Autodesk Fusion 360 part; units mm, degrees
note: some values were not read from the file. Set by a fixed rule: which sketch regions a step uses.
(part 2 of 2)
extrude "Extruir44" add sketch "Boceto37" along normal blind 1 bodies 7
mirror "Simetría3" about plane through (0, 238.5, 45.4) normal (1, 0, 0) of bodies 7 merged
sketch "Boceto38" plane through (0, 266.5, 0) normal (0, 1, 0) x (-1, 0, 0)
  line L0 (-75, 1.5333) -> (-75, 8.4667)
  line L1 (-75, 8.4667) -> (-88.0667, 8.4667)
  line L2 (-88.0667, 8.4667) -> (-88.0667, 1.5333)
  line L3 (-88.0667, 1.5333) -> (-75, 1.5333)
sketch "Boceto44" plane through (88.0667, 0, 0) normal (1, 0, 0) x (0, 1, 0)
  line L0 (189.5, 8.4667) -> (189.5, 1.5333)
  line L1 (189.5, 1.5333) -> (266.5, 1.5333)
  line L2 (266.5, 1.5333) -> (266.5, 8.4667)
  line L3 (266.5, 8.4667) -> (189.5, 8.4667)
  line L4 (266.5, 8.4667) -> (184.5, 8.4667)
  line L5 (184.5, 8.4667) -> (184.5, 7.9667)
  line L6 (184.5, 7.9667) -> (266.5, 7.9667)
  line L7 (266.5, 7.9667) -> (266.5, 8.4667)
  line L8 (266.5, 1.5333) -> (184.5, 1.5333)
  line L9 (184.5, 1.5333) -> (184.5, 2.0333)
  line L10 (184.5, 2.0333) -> (266.5, 2.0333)
  line L11 (266.5, 2.0333) -> (266.5, 1.5333)
  dimension "d231" = 82
  dimension "d232" = 0.5
  dimension "d233" = 82
  dimension "d234" = 0.5
  constraint horizontal L4
  constraint vertical L5
  constraint horizontal L6
  constraint vertical L7
  constraint coincident L2.end L3.start
  constraint horizontal L8
  constraint vertical L9
  constraint horizontal L10
  constraint vertical L11
  constraint coincident L1.end L2.start
  measures "d231" distance of L2.end L4.end
  measures "d232" distance of L2.end L6.end
  measures "d233" distance of L1.end L8.end
  measures "d234" distance of L1.end L10.end
extrude "Extruir48" cut sketch "Boceto44" against normal blind 13.067 contours L0 L2 L3 L4 L6 L7 | L0 L4 L5 L6 | L0 L1 L2 L8 L10 L11 | L0 L8 L9 L10 bodies 3
sketch "Boceto45" plane through (-88.0667, 0, 0) normal (-1, 0, 0) x (0, -1, 0)
  line L0 (-189.5, 1.5333) -> (-189.5, 8.4667)
  line L1 (-189.5, 8.4667) -> (-266.5, 8.4667)
  line L2 (-266.5, 8.4667) -> (-266.5, 1.5333)
  line L3 (-266.5, 1.5333) -> (-189.5, 1.5333)
  line L4 (-266.5, 1.5333) -> (-184.5, 1.5333)
  line L5 (-184.5, 1.5333) -> (-184.5, 2.0333)
  line L6 (-184.5, 2.0333) -> (-266.5, 2.0333)
  line L7 (-266.5, 2.0333) -> (-266.5, 1.5333)
  line L8 (-266.5, 8.4667) -> (-184.5, 8.4667)
  line L9 (-184.5, 8.4667) -> (-184.5, 7.9667)
  line L10 (-184.5, 7.9667) -> (-266.5, 7.9667)
  line L11 (-266.5, 7.9667) -> (-266.5, 8.4667)
  dimension "d237" = 82
  dimension "d238" = 0.5
  dimension "d239" = 82
  dimension "d240" = 0.5
  constraint horizontal L4
  constraint vertical L5
  constraint horizontal L6
  constraint vertical L7
  constraint coincident L2.end L3.start
  constraint horizontal L8
  constraint vertical L9
  constraint horizontal L10
  constraint vertical L11
  constraint coincident L1.end L2.start
  measures "d237" distance of L2.end L4.end
  measures "d238" distance of L2.end L6.end
  measures "d239" distance of L1.end L8.end
  measures "d240" distance of L1.end L10.end
extrude "Extruir49" cut sketch "Boceto45" against normal blind 13.067 contours L0 L2 L3 L4 L6 L7 | L0 L4 L5 L6 | L0 L1 L2 L8 L10 L11 | L0 L8 L9 L10 bodies 3
sketch "Boceto46" plane through (88.0667, 0, 0) normal (1, 0, 0) x (0, 1, 0)
  line L0 (266.5, 7.9667) -> (189.5, 7.9667)
  line L1 (189.5, 7.9667) -> (189.5, 2.0333)
  line L2 (189.5, 2.0333) -> (266.5, 2.0333)
  line L3 (266.5, 2.0333) -> (266.5, 7.9667)
  line L4 (266.5, 7.9667) -> (184, 7.9667)
  line L5 (184, 7.9667) -> (184, 2.0333)
  line L6 (184, 2.0333) -> (266.5, 2.0333)
  line L7 (266.5, 2.0333) -> (266.5, 7.9667)
  dimension "d243" = 82.5
  constraint horizontal L4
  constraint vertical L5
  constraint horizontal L6
  constraint vertical L7
  constraint coincident L0.start L3.end
  measures "d243" distance of L0.start L4.end
extrude "Extruir50" [suppressed]
sketch "Boceto47" plane through (-88.0667, 0, 0) normal (-1, 0, 0) x (0, -1, 0)
  line L0 (-266.5, 2.0333) -> (-189.5, 2.0333)
  line L1 (-189.5, 2.0333) -> (-189.5, 7.9667)
  line L2 (-189.5, 7.9667) -> (-266.5, 7.9667)
  line L3 (-266.5, 7.9667) -> (-266.5, 2.0333)
  line L4 (-266.5, 7.9667) -> (-184, 7.9667)
  line L5 (-184, 7.9667) -> (-184, 2.0333)
  line L6 (-184, 2.0333) -> (-266.5, 2.0333)
  line L7 (-266.5, 2.0333) -> (-266.5, 7.9667)
  dimension "d246" = 82.5
  constraint horizontal L4
  constraint vertical L5
  constraint horizontal L6
  constraint vertical L7
  constraint coincident L2.end L3.start
  measures "d246" distance of L2.end L4.end
extrude "Extruir51" [suppressed]
equation "d3 = Altura_Columna"
equation "Altura_Columna = 200 mm"
equation "Ancho_Estructura = 10 mm"
equation "Espesor_Columna = 1 mm"
equation "d11 = Espesor_Columna"
equation "d12 = d13"
equation "d14 = d13"
equation "d15 = d16"
equation "d17 = d16"
equation "d18 = Ancho_Estructura"
equation "d34 = Ancho_Estructura + ( 0.4 * 2 ) * 1 mm + 5 mm"
equation "d38 = -( Ancho_Estructura + 0.8 mm )"
equation "d109 = -Altura_Columna - 70 mm"
equation "d153 = Ancho_Columna"
equation "Ancho_Columna = 9.99 mm"
equation "d155 = Espesor_Columna * -1"
equation "d164 = Ancho_Estructura * -3"
named bodies: "PColumna", "Base Inferior", "Base Superior", "Cilindro", "Carril Derecho", "Carril Izquierdo", "Complemento"
